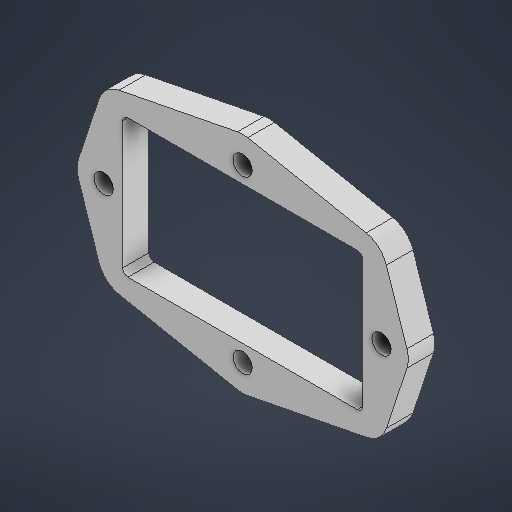
# Autodesk Inventor part: Clamp
Saved by Autodesk Inventor 2026.1 (Build 301233000, 233)
## iProperties
Created: 2025-09-03
Part Number: Clamp
Material: Generic
Document SubType Name: Modeling
Designer: Teddy
Density: 1 g/cm^3
Appearance: Default
Author: Teddy
Autodesk Inventor part; units mm, degrees
ref_plane "Work Plane1" through (0, 20.5423, 0) normal (0, 0, 1) x (-1, 0, 0)
sketch "Sketch1" plane through (0, 20.5423, 0) normal (0, 0, 1) x (-1, 0, 0)
  line L0 (-25.854, -3.81) -> (40.186, -3.81) construction
  line L1 (40.186, -3.81) -> (40.186, 36.83) construction
  line L2 (40.186, 36.83) -> (-25.854, 36.83) construction
  line L3 (-25.854, 36.83) -> (-25.854, -3.81) construction
  line L4 (-19.9104, 0) -> (34.2424, 0) projected
  line L5 (35.8299, 1.5875) -> (35.8299, 31.4325) projected
  line L6 (34.2424, 33.02) -> (-19.9104, 33.02) projected
  line L7 (-21.4979, 31.4325) -> (-21.4979, 1.5875) projected
  line L8 (7.166, 0) -> (7.166, 33.02)
  line L9 (-21.4979, 16.51) -> (35.8299, 16.51)
  circle A0 centre (7.166, -3.81) radius 2.286
  circle A1 centre (40.186, 16.51) radius 2.286
  circle A2 centre (7.166, 36.83) radius 2.286
  circle A3 centre (-25.854, 16.51) radius 2.286
  arc A4 (-31.886, 18.4944) -> (-31.886, 14.5256) centre (-25.854, 16.51) ccw
  arc A5 (8.3871, 43.0615) -> (5.9448, 43.0615) centre (7.166, 36.83) ccw
  arc A6 (46.218, 14.5256) -> (46.218, 18.4944) centre (40.186, 16.51) ccw
  arc A7 (5.9448, -10.0415) -> (13.516, -3.81) centre (7.166, -3.81) ccw
  line L10 (8.3871, -10.0415) -> (40.186, -3.81)
  line L11 (40.186, -3.81) -> (46.218, 14.5256)
  line L12 (46.218, 18.4944) -> (40.186, 36.83)
  line L13 (40.186, 36.83) -> (8.3871, 43.0615)
  line L14 (5.9448, 43.0615) -> (-25.854, 36.83)
  line L15 (-25.854, 36.83) -> (-31.886, 18.4944)
  line L16 (-31.886, 14.5256) -> (-25.854, -3.81)
  line L17 (-25.854, -3.81) -> (5.9448, -10.0415)
  arc A8 (0.816, -3.81) -> (5.9448, -10.0415) centre (7.166, -3.81) ccw
  arc A9 (13.516, -3.81) -> (0.816, -3.81) centre (7.166, -3.81) ccw construction
  arc A10 (40.186, 10.16) -> (46.218, 14.5256) centre (40.186, 16.51) ccw
  arc A11 (46.218, 18.4944) -> (40.186, 10.16) centre (40.186, 16.51) ccw construction
  arc A12 (13.516, 36.83) -> (8.3871, 43.0615) centre (7.166, 36.83) ccw
  arc A13 (5.9448, 43.0615) -> (13.516, 36.83) centre (7.166, 36.83) ccw construction
  arc A14 (-25.854, 22.86) -> (-31.886, 18.4944) centre (-25.854, 16.51) ccw construction
  arc A15 (-31.886, 14.5256) -> (-25.854, 22.86) centre (-25.854, 16.51) ccw construction
  point P0 (0, 20.5423)
  dimension "d0" = 20.32
  dimension "d1" = 33.02
  dimension "d2" = 20.32
  dimension "d3" = 33.02
  dimension "d4" = 4.572
  dimension "d5" = 4.572
  dimension "d6" = 4.572
  dimension "d7" = 4.572
  dimension "d8" = 12.7
  dimension "d9" = 12.7
  dimension "d10" = 12.7
  dimension "d11" = 12.7
  constraints: 28 end point, 26 point on circle, 16 centre point, 12 tangent, 8 midpoint, 5 point on line, 4 coincident, 4 parallel, 1 horizontal, 1 perpendicular
  measures "d0" distance between parallel lines of L0 L9
  measures "d1" distance between parallel lines of L3 L8
  measures "d2" distance between parallel lines of L9 L2
  measures "d3" distance between parallel lines of L8 L1
  measures "d4" diameter of A0
  measures "d5" diameter of A1
  measures "d6" diameter of A2
  measures "d7" diameter of A3
  measures "d8" diameter of A4
  measures "d9" diameter of A5
  measures "d10" diameter of A6
  measures "d11" diameter of A7
extrude "Extrusion1" add sketch "Sketch1" along normal blind 6.35
fillet "Fillet1" radius 6.35 4 edges at (25.854, 24.3523, 3.175) (-40.186, 24.3523, 3.175) (-40.186, -16.2877, 3.175) (25.854, -16.2877, 3.175)
ref_plane "Work Plane2" through (-35.4607, 20.5423, 21.1505) normal (-0.9998477, 0, 0.0174524) x (-0.0174524, 0, -0.9998477)
sketch "Sketch2" plane through (-35.4607, 20.5423, 21.1505) normal (-0.9998477, 0, 0.0174524) x (-0.0174524, 0, -0.9998477)
  line L0 (-20.4302, 2.313) -> (-20.4302, 30.707) projected
  line L1 (21.1537, 1.5873) -> (-20.4302, 2.313) projected
  line L2 (21.1537, 1.5873) -> (21.1537, 1.5875) projected
  line L3 (21.1537, 31.4325) -> (21.1537, 31.4327) projected
  line L4 (-20.4302, 30.707) -> (21.1537, 31.4327) projected
  line L5 (-20.4579, 0.7257) -> (21.126, 0) projected
  line L6 (21.126, 33.02) -> (-20.4579, 32.2943) projected
  line L7 (14.3044, 34.544) -> (20.6534, 34.544) projected
  line L8 (-20.4579, 0.7257) -> (-20.4579, 32.2943)
  line L9 (35.4438, -3.9898) -> (35.4438, 36.1843)
  line L10 (-20.4579, 0.7257) -> (35.4438, -0.2499)
  line L11 (-20.4579, 32.2943) -> (35.4438, 33.298)
  point P0 (20.5284, 20.5423)
  point P1 (21.126, 0)
  constraints: 8 end point, 3 point on line, 1 vertical
ref_plane "Work Plane3" through (21.4977, -10.8904, 0.0127) normal (0.9998477, 0, 0.0174524) x (0, 1, 0)
extrude "Extrusion2" add sketch "Sketch2" against normal up to surface separate body surface through (21.4977, -10.8904, 0.0127) normal (0.9998477, 0, 0.0174524)
fillet "Fillet2" radius 1.27 6 edges at (21.1518, 20.1795, 19.8282) (21.6399, 20.6673, -8.1354) (-35.9543, 20.6673, -7.1301) (-35.4665, 20.1795, 20.8165) (-35.5915, -12.2538, 13.6587) (21.2768, -12.2538, 12.6661)
combine bodies "Combine1" operation type subtract main body 1 bodies to subtract 2
body "Solid1"
